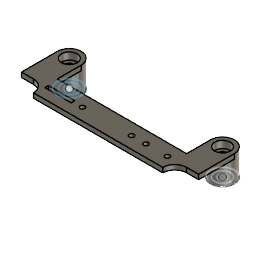
Support_capteur_boite (Autodesk Fusion 360 design; units mm, degrees)
Autodesk Fusion 360 part; units mm, degrees
note: some values were not read from the file. Set by a fixed rule: which sketch regions a step uses.
sketch "Esquisse1" plane through (0, 0, 0) normal (0, 0, 1) x (1, 0, 0)
  circle A0 centre (0, 0) radius 5
  circle A1 centre (0, 0) radius 3.25
  circle A2 centre (-64, 0) radius 3.25
  circle A3 centre (-64, 0) radius 5
  circle A4 centre (-64, 0) radius 1.75
  circle A5 centre (0, 0) radius 1.75
  dimension "d1" = 10
  dimension "d2" = 6.5
  dimension "d3" = 6.5
  dimension "d4" = 64
  dimension "d5" = 10
  dimension "d6" = 3.5
  dimension "d7" = 3.5
  constraint coincident A0.centre A1.centre
  constraint concentric A0 A1
  constraint concentric A2 A3
  constraint concentric A3 A4
  constraint concentric A1 A5
  measures "d1" diameter of A0
  measures "d2" diameter of A1
  measures "d3" diameter of A2
  measures "d4" distance of A0.centre A2.centre
  measures "d5" diameter of A3
  measures "d6" diameter of A4
  measures "d7" diameter of A5
extrude "Extrusion1" add sketch "Esquisse1" along normal blind 11 contours A0 | A3 makes body 1 at (4.9938, -0.2492, 7.3333) makes body 2 at (-59.0062, -0.2492, 7.3333)
extrude "Extrusion2" add sketch "Esquisse1" along normal blind 8 contours A1 | A2 bodies 1 2
sketch "Esquisse5" plane through (0, 0, 11) normal (0, 0, 1) x (-1, 0, 0)
  circle A0 centre (64, 0) radius 3.25
  circle A1 centre (64, 0) radius 5
  line L0 (69, 0.0096) -> (69, 15)
  line L1 (64, 20) -> (5, 20)
  line L2 (-5, 15) -> (-5, 0.0071)
  line L3 (59, 0) -> (59, 10)
  line L4 (59, 10) -> (5, 10)
  line L5 (5, 10) -> (5, 0.0071)
  circle A2 centre (0, 0) radius 5
  arc A3 (59, 20) -> (64, 15) centre (64, 20) ccw
  line L6 (64, 20) -> (64, 15) construction
  line L7 (64, 15) -> (69, 15)
  arc A4 (0, 15) -> (5, 20) centre (0, 20) ccw
  line L8 (0, 20) -> (0, 15) construction
  line L9 (0, 20) -> (5, 20) construction
  line L10 (0, 15) -> (-5, 15)
  dimension "d35" = 5
  dimension "d37" = 5
  dimension "d38" = 5
  dimension "d39" = 90
  dimension "d40" = 5
  constraint coincident A1 L0.start
  constraint vertical L0
  constraint perpendicular L0 L1
  constraint coincident L2.end A2
  constraint coincident L1 A3.start
  constraint tangent A3 L7
  constraint tangent A4 L10
  constraint perpendicular L2 L10
  measures "d35" radius of A3
  measures "d37" distance of L0 L1.start
  measures "d38" radius of A4
  measures "d39" angle of L8 L9
  measures "d40" distance of L2 A4.centre
extrude "Extrusion3" add sketch "Esquisse5" against normal blind 2 contours A1 L0 L1 L2 L3 L4 L5 A2 A3 L7 A4 L10 bodies 1 2
sketch "Esquisse6" plane through (0, 0, 11) normal (0, 0, 1) x (-1, 0, 0)
  circle A0 centre (64, 0) radius 3.25
  circle A1 centre (0, 0) radius 3.25
  arc A2 (-5, 0.0071) -> (5, 0) centre (0, 0) ccw
  line L0 (5, 0.0071) -> (5, 10)
  line L1 (5, 10) -> (59, 10)
  line L2 (59, 10) -> (59, 0)
  arc A3 (59, 0) -> (69, 0) centre (64, 0) ccw
  line L3 (69, 0.0096) -> (69, 15)
  line L4 (59, 20) -> (5, 20)
  line L5 (-5, 15) -> (-5, 0.0071)
  circle A4 centre (8, 15) radius 1
  circle A5 centre (17, 15) radius 1
  circle A6 centre (23, 15) radius 1
  circle A7 centre (43.5, 15) radius 1
  line L6 (47.5, 15) -> (47.5, 15.75)
  line L7 (47.5, 15.75) -> (58.5, 15.75)
  line L8 (58.5, 15.75) -> (58.5, 14.25)
  line L9 (58.5, 14.25) -> (47.5, 14.25)
  line L10 (47.5, 14.25) -> (47.5, 15)
  line L11 (69, 15) -> (64, 15)
  arc A8 (59, 20) -> (64, 15) centre (64, 20) ccw
  arc A9 (0, 15) -> (5, 20) centre (0, 20) ccw
  line L12 (0, 15) -> (-5, 15)
  dimension "d20" = 2
  dimension "d21" = 3
  dimension "d22" = 5
  dimension "d23" = 2
  dimension "d24" = 9
  dimension "d25" = 2
  dimension "d26" = 6
  dimension "d27" = 2
  dimension "d28" = 20.5
  dimension "d29" = 0.75
  dimension "d30" = 11
  dimension "d31" = 4
  dimension "d32" = 1.5
  constraint vertical L6
  constraint perpendicular L6 L7
  constraint perpendicular L7 L8
  constraint perpendicular L6 L9
  constraint perpendicular L9 L10
  measures "d20" diameter of A4
  measures "d21" distance of L0 A4.centre
  measures "d22" distance of L1 A4.centre
  measures "d23" diameter of A5
  measures "d24" distance of A4.centre A5.centre
  measures "d25" diameter of A6
  measures "d26" distance of A5.centre A6.centre
  measures "d27" diameter of A7
  measures "d28" distance of A6.centre A7.centre
  measures "d29" distance of L6.start L6.end
  measures "d30" distance of L6.end L7.end
  measures "d31" distance of A7.centre L6.start
  measures "d32" distance of L7.end L8.end
extrude "Extrusion4" cut sketch "Esquisse6" against normal up to surface (2 mm away) contours A4 | A5 | A6 | A7 | L6 L7 L8 L9 L10 bodies 1
